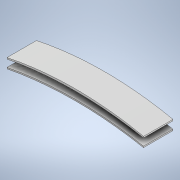
# Autodesk Inventor part: arc_de_cercle
Saved by Autodesk Inventor 2020.2 (Build 242310000, 310)
## iProperties
Created: 2020-01-28
Part Number: arc_de_cercle
Material: Générique
Document SubType Name: Modeling
Designer: anton
Density: 1 g/cm^3
Appearance: Par défaut
Author: anton
Autodesk Inventor part; units mm, degrees
ref_plane "YZ Plane" through (0, 0, 0) normal (1, 0, 0) x (0, 1, 0)
ref_plane "XZ Plane" through (0, 0, 0) normal (0, 1, 0) x (-1, 0, 0)
ref_plane "XY Plane" through (0, 0, 0) normal (0, 0, 1) x (1, 0, 0)
sketch "Esquisse1" plane through (0, 0, 0) normal (0, 0, 1) x (1, 0, 0)
  line L0 (-150.5839, 785.7) -> (150.5839, 785.7)
  arc A0 (150.5839, 785.7) -> (-150.5839, 785.7) centre (0, 0) ccw
  line L1 (-150.5839, 801.4) -> (150.5839, 801.4)
  arc A1 (150.5839, 801.4) -> (-150.5839, 801.4) centre (0, 15.7) ccw
  line L2 (-150.5839, 782.7) -> (150.5839, 782.7)
  line L3 (-150.5839, 804.4) -> (150.5839, 804.4)
  line L4 (0, 797) -> (-150.5839, 797)
  arc A2 (150.5839, 782.7) -> (-150.5839, 782.7) centre (0, -3) ccw
  line L5 (0, 820.1) -> (-146.2821, 820.1)
  arc A3 (150.5839, 804.4) -> (-150.5839, 804.4) centre (0, 90.1) ccw
  line L6 (-150.5839, 804.4) -> (-150.5839, 801.4)
  line L7 (-150.5839, 785.7) -> (-150.5839, 782.7)
  line L8 (150.5839, 804.4) -> (150.5839, 801.4)
  line L9 (150.5839, 785.7) -> (150.5839, 782.7)
  point P0 (0, 0)
  dimension "d4" = 785.7
  dimension "d6" = 15.7
  dimension "d7" = 3
  dimension "d8" = 3
  dimension "d9" = 14.3
  dimension "d10" = 15.7
  constraints: 20 end point, 10 point on circle, 6 horizontal, 4 centre point, 1 collinear, 1 perpendicular, 1 vertical
  measures "d4" distance from line of point (0, 0) L0
  measures "d6" distance between parallel lines of L0 L1
  measures "d7" distance between parallel lines of L1 L3
  measures "d8" distance between parallel lines of L0 L2
  measures "d9" distance between parallel lines of L2 L4
  measures "d10" distance between parallel lines of L3 L5
extrude "Extrusion1" add sketch "Esquisse1" along normal blind 65 contours A0 L4 A2 L0 | L0 A2 L7 | A0 L0 A2 L4 | L0 L9 A2 | L6 L3 A1 | A1 L3 L8 | L3 A3 A1
